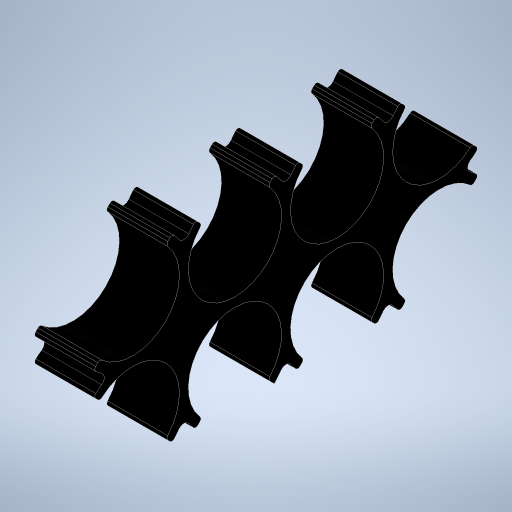
# Autodesk Inventor part: BatterieClamp
Saved by Autodesk Inventor 2024 (Build 280153000, 153)
## iProperties
Created: 2023-12-27
Part Number: BatterieClamp
Material: Generisch
Document SubType Name: Modeling
Designer: denni
Density: 1 g/cm^3
Appearance: Vorgabe(1)
Author: denni
Autodesk Inventor part; units mm, degrees
ref_plane "YZ Plane" through (0, 0, 0) normal (1, 0, 0) x (0, 1, 0)
ref_plane "XZ Plane" through (0, 0, 0) normal (0, 1, 0) x (-1, 0, 0)
ref_plane "XY Plane" through (0, 0, 0) normal (0, 0, 1) x (1, 0, 0)
sketch "Skizze2" plane through (0, 0, 0) normal (1, 0, 0) x (0, 1, 0)
  circle A0 centre (0, 0) radius 7.75
  circle A1 centre (0, 0) radius 8.5
  circle A2 centre (0, 0) radius 9.25
  line L0 (0, 0) -> (9.25, 0) construction
  line L1 (0, 0) -> (0, -9.25) construction
  line L2 (-6.5407, 6.5407) -> (6.5407, -6.5407)
  line L3 (-6.5407, -6.5407) -> (6.5407, 6.5407)
  circle A3 centre (0, -17) radius 7.75
  circle A4 centre (0, -17) radius 8.5
  circle A5 centre (0, -17) radius 9.25
  line L4 (-6.5407, -23.5407) -> (6.5407, -10.4593)
  line L5 (-6.5407, -10.4593) -> (6.5407, -23.5407)
  circle A6 centre (0, -34) radius 7.75
  circle A7 centre (0, -34) radius 8.5
  circle A8 centre (0, -34) radius 9.25
  line L6 (-6.5407, -40.5407) -> (6.5407, -27.4593)
  line L7 (-6.5407, -27.4593) -> (6.5407, -40.5407)
  circle A9 centre (0, -51) radius 7.75
  circle A10 centre (0, -51) radius 8.5
  circle A11 centre (0, -51) radius 9.25
  line L8 (-6.5407, -57.5407) -> (6.5407, -44.4593)
  line L9 (-6.5407, -44.4593) -> (6.5407, -57.5407)
  circle A12 centre (17, 0) radius 7.75
  circle A13 centre (17, 0) radius 8.5
  circle A14 centre (17, 0) radius 9.25
  line L10 (10.4593, -6.5407) -> (23.5407, 6.5407)
  line L11 (10.4593, 6.5407) -> (23.5407, -6.5407)
  circle A15 centre (17, -17) radius 7.75
  circle A16 centre (17, -17) radius 8.5
  circle A17 centre (17, -17) radius 9.25
  line L12 (10.4593, -23.5407) -> (23.5407, -10.4593)
  line L13 (10.4593, -10.4593) -> (23.5407, -23.5407)
  circle A18 centre (17, -34) radius 7.75
  circle A19 centre (17, -34) radius 8.5
  circle A20 centre (17, -34) radius 9.25
  line L14 (10.4593, -40.5407) -> (23.5407, -27.4593)
  line L15 (10.4593, -27.4593) -> (23.5407, -40.5407)
  circle A21 centre (17, -51) radius 7.75
  circle A22 centre (17, -51) radius 8.5
  circle A23 centre (17, -51) radius 9.25
  line L16 (10.4593, -57.5407) -> (23.5407, -44.4593)
  line L17 (10.4593, -44.4593) -> (23.5407, -57.5407)
  point P0 (9.25, -17)
  point P1 (0, -26.25)
  point P2 (9.25, -34)
  point P3 (0, -43.25)
  point P4 (9.25, -51)
  point P5 (0, -60.25)
  point P6 (26.25, 0)
  point P7 (17, -9.25)
  point P8 (26.25, -17)
  point P9 (17, -26.25)
  point P10 (26.25, -34)
  point P11 (17, -43.25)
  point P12 (26.25, -51)
  point P13 (17, -60.25)
  point P14 (-5.4801, -5.4801)
  point P15 (-3.6486, -8.5)
  point P16 (-5.4801, -11.5199)
  point P17 (-5.4801, -22.4801)
  point P18 (-3.6486, -25.5)
  point P19 (-5.4801, -28.5199)
  point P20 (-5.4801, -39.4801)
  point P21 (-3.6486, -42.5)
  point P22 (-5.4801, -45.5199)
  point P23 (5.4801, -56.4801)
  point P24 (8.5, -54.6486)
  point P25 (11.5199, -56.4801)
  point P26 (22.4801, -45.5199)
  point P27 (20.6486, -42.5)
  point P28 (22.4801, -39.4801)
  point P29 (22.4801, -28.5199)
  point P30 (20.6486, -25.5)
  point P31 (22.4801, -22.4801)
  point P32 (22.4801, -11.5199)
  point P33 (20.6486, -8.5)
  point P34 (22.4801, -5.4801)
  point P35 (11.5199, 5.4801)
  point P36 (8.5, 3.6486)
  point P37 (5.4801, 5.4801)
  dimension "d13" = 15.5
  dimension "a" = 17
  dimension "d15" = 18.5
  dimension "d16" = 45
  dimension "d19" = 17
  dimension "d22" = 17
  constraints: 40 point on circle, 36 end point, 24 centre point, 18 coincident, 2 horizontal, 2 midpoint, 2 perpendicular, 1 vertical, 105 other
  measures "d13" diameter of A0
  measures "a" diameter of A1
  measures "d15" diameter of A2
  measures "d16" angle of L1 L2
  measures "d19" distance of A0.centre A3.centre
  measures "d22" distance of A0.centre A12.centre
extrude "Extrusion1" add sketch "Skizze2" along normal blind 10 contours A14 A1 L2 A0 | A0 L3 A1 A14 | A14 A1 | L2 A1 A5 A0 | A14 A2 A13 A1 | A1 L3 A2 A14 | A14 A2 L2 A1 | A1 A13 A2 A14 | A5 A1 L3 A0 | A5 A1 | L2 A2 A5 A1 | A13 A2 | A14 L11 A13 A2 | A14 A17 A5 A2 | A2 A13 L10 A14 | A5 A2 A4 A1 | A5 A2 L3 A1 | A1 A4 A2 A5 | A13 L11 A12 A2 | A2 A12 L10 A13 | L10 A13 A17 A14 | A4 A2 | A5 L4 A4 A2 | A2 A4 L5 A5 | L10 A12 A17 A13 | A17 A13 A16 A14 | A14 A16 L13 A17 | A4 L4 A3 A2 | A2 A3 L5 A4 | A5 A17 A4 L4 | A17 A13 | A16 A14 | A14 A15 L13 A16 | L13 A16 A5 A17 | A4 A17 A3 L4 | A5 A16 A4 A17 | L4 A4 A8 A5 | A12 L11 A13 A17 | A13 A17 A14 A16 | A14 A17 A13 L11 | A14 A16 L12 A15 | L13 A15 A5 A16 | A4 A17 | L4 A3 A8 A4 | A5 A16 | A8 A4 A7 A5 | A5 A7 L7 A8 | A14 A17 L12 A16 | A17 A4 L5 A3 | A16 A5 A17 A4 | A8 A4 | A15 L12 A16 A5 | A7 A5 | A5 A6 L7 A7 | L5 A4 A8 A3 | A17 A5 L5 A4 | A16 L12 A17 A5 | A4 A8 A5 A7 | A15 A20 A16 L12 | A5 A7 L6 A6 | L6 A7 A11 A8 | L13 A16 A20 A15 | L5 A5 A8 A4 | A17 A20 A8 A5 | A16 A20 A17 L12 | A5 A8 L6 A7 | A20 A16 | L6 A7 A20 A6 | L6 A6 A11 A7 | A11 A7 A10 A8 | A8 A10 L9 A11 | L13 A17 A20 A16 | A16 A19 A17 A20 | L6 A8 A20 A7 | A20 A17 A19 A16 | A20 A7 L7 A6 | A20 A7 | A11 A7 | A10 A8 | A8 A9 L9 A10 | A20 L14 A19 A17 | A17 A19 L15 A20 | A19 A17 | A20 A8 A19 A7 | L7 A7 A11 A6 | A20 A8 L7 A7 | A7 A19 A8 A20 | A7 A11 A8 A10 | A8 A10 L8 A9 | A19 L14 A18 A17 | A17 A18 L15 A19 | L15 A19 A8 A20 | A19 A8 | L7 A8 A11 A7 | A20 A23 A11 A8 | A8 A19 L14 A20 | A8 A11 L8 A10 | L8 A10 A23 A9 | L9 A10 A23 A11 | L15 A18 A8 A19 | A8 A18 L14 A19 | L14 A19 A23 A20 | L8 A11 A23 A10 | A23 A10 L9 A9 | A23 A10 | A23 A10 A22 A11 | A11 A22 L16 A23 | A20 A23 A19 L15 | L14 A18 A23 A19 | A23 A19 A22 A20 | A20 A22 L17 A23 | A23 A11 A22 A10 | A22 A11 | A11 A21 L16 A22 | A19 A23 A18 L15 | A23 L16 A22 A20 | A20 A22 A19 A23 | A23 A19 | A22 A20 | A20 A21 L17 A22 | L17 A22 A11 A23 | A11 A22 L17 A21 | A22 L16 A21 A20
fillet "Rundung1" radius 1 8 edges at (5, 20.6486, -8.5) (5, 8.5, 3.6486) (5, -3.6486, -8.5) (5, -3.6486, -25.5) (5, -3.6486, -42.5) (5, 8.5, -54.6486) (5, 20.6486, -42.5) (5, 20.6486, -25.5)
fillet "Rundung2" radius 0.5 31 edges at (5, 10.4593, 6.5407) (5, 11.5199, 5.4801) (5, 22.4801, -5.4801) (5, 23.5407, -6.5407) (5, 23.5407, -10.4593) (5, 22.4801, -11.5199) (5, 22.4801, -22.4801) (5, 23.5407, -23.5407) (5, 23.5407, -27.4593) (5, 22.4801, -28.5199) (5, 22.4801, -39.4801) (5, 23.5407, -40.5407) (5, 23.5407, -44.4593) (5, 22.4801, -45.5199) (5, 11.5199, -56.4801) (5, 10.4593, -57.5407) (5, 6.5407, -57.5407) (5, 5.4801, -56.4801) (5, -5.4801, -45.5199) (5, -6.5407, -44.4593) (5, -6.5407, -40.5407) (5, -5.4801, -39.4801) (5, -5.4801, -28.5199) (5, -6.5407, -27.4593) (5, -5.4801, -22.4801) (5, -5.4801, -11.5199) (5, -6.5407, -10.4593) (5, -6.5407, -6.5407) (5, -5.4801, -5.4801) (5, 6.5407, 6.5407) (5, 5.4801, 5.4801)
equation "\"d19\" = a"
equation "\"d22\" = a"
